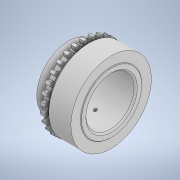
# Autodesk Inventor part: 73. Шестерня третьей передачи
Saved by Autodesk Inventor 2021 (Build 250183000, 183)
## iProperties
Created: 2021-03-26
Part Number: 73. Шестерня третьей передачи
Material: Типовые
Document SubType Name: Modeling
Designer: Данил
Density: 1 g/cm^3
Appearance: По умолчанию
Author: Данил
Autodesk Inventor part; units mm, degrees
ref_plane "YZ Plane" through (0, 0, 0) normal (1, 0, 0) x (0, 1, 0)
sketch "Эскиз1" plane through (0, 0, 0) normal (0, 0, 1) x (1, 0, 0)
  line L0 (-21.5, 0) -> (21.5, 0)
  line L1 (-21.5, -31.5) -> (-10.9, -32)
  line L2 (-21.5, -31.5) -> (-21.5, -25.6)
  line L3 (-19.9, -24) -> (19.9, -24)
  line L4 (-19.9, -24) -> (-21.5, -25.6)
  line L5 (-10.9, -32) -> (-10.9, -32)
  line L6 (-10.4, -31.5) -> (-10.4, -31.5)
  line L7 (-9.9, -32) -> (-9.9, -40.5)
  arc A0 (-10.4, -31.5) -> (-10.9, -32) centre (-10.4, -32) ccw
  arc A1 (-9.9, -32) -> (-10.4, -31.5) centre (-10.4, -32) ccw
  line L8 (-9.9, -40.5) -> (-4.4, -40.5)
  line L9 (-4.4, -40.5) -> (-4.4, -36.5)
  line L10 (-4.4, -36.5) -> (-1, -36.5)
  line L11 (-1, -36.5) -> (-1, -49.276)
  line L12 (-1, -49.276) -> (21, -49.276)
  line L13 (21, -49.276) -> (21, -30.5)
  line L14 (21.5, -30) -> (21.5, -30)
  line L15 (21.5, -30) -> (21.5, -25.6)
  arc A2 (21.5, -30) -> (21, -30.5) centre (21.5, -30.5) ccw
  line L16 (19.9, -24) -> (21.5, -25.6)
  point P0 (0, 0)
  point P1 (0, 0)
  point P2 (-21.5, -24)
  point P3 (21.5, -24)
  dimension "d0" = 43
  dimension "d1" = 1.6
  dimension "d2" = 45
  dimension "d3" = 48
  dimension "d6" = 63
  dimension "d7" = 64
  dimension "d8" = 1
  dimension "d9" = 0.5
  dimension "d10" = 63
  dimension "d11" = 32.4
  dimension "d12" = 5.5
  dimension "d13" = 3.4
  dimension "d14" = 22
  dimension "d17" = 81
  dimension "d18" = 73
  dimension "d19" = 98.552
  dimension "d20" = 0.5
  dimension "d21" = 60
  dimension "d22" = 1.6
  dimension "d23" = 45
  constraints: 34 end point, 7 perpendicular, 6 point on circle, 6 tangent, 4 horizontal, 4 point on line, 3 centre point, 3 vertical, 2 vertical alignment, 1 coincident, 1 concentric, 1 midpoint
  measures "d0" distance of L0.start L0.end
  measures "d1" distance of L3.start point (-21.5, -24)
  measures "d2" angle of L3 L4
  measures "d3" diameter of L3 L0
  measures "d6" diameter of L1.start L0
  measures "d7" diameter of L1.end L0
  measures "d8" distance between parallel lines of L5 L7
  measures "d9" radius of A0
  measures "d10" diameter of L6 L0
  measures "d11" horizontal distance of L0.end L1.end
  measures "d12" distance between parallel lines of L7 L9
  measures "d13" distance of L9.end L10.end
  measures "d14" distance of L11.end L12.end
  measures "d17" diameter of L8 L0
  measures "d18" diameter of L10 L0
  measures "d19" diameter of L12 L0
  measures "d20" radius of A2
  measures "d21" diameter of L14.end L0
  measures "d22" distance of L3.end point (21.5, -24)
  measures "d23" angle of L3 L16
revolve "Вращение1" add sketch "Эскиз1" angle 360 about axis through (-21.5, 0, 0) along (1, 0, 0)
sketch "Эскиз2" plane through (-9.9, 0, 0) normal (-1, 0, 0) x (0, 0, 1)
  circle A0 centre (0, 0) radius 40.5 projected
  circle A1 centre (0, 0) radius 39 construction
  circle A2 centre (0, 0) radius 37
  arc A3 (-1.515, 40.4717) -> (-2.077, 36.9417) centre (3.6162, 37.8449) ccw
  arc A4 (2.077, 36.9417) -> (1.515, 40.4717) centre (-3.6162, 37.8449) ccw
  line L0 (-2.042, 38.9465) -> (2.042, 38.9465) construction
  line L1 (-1.515, 40.4717) -> (1.515, 40.4717) construction
  arc A5 (-9.8964, 39.2723) -> (-9.7123, 35.7026) centre (-4.3312, 37.7697) ccw
  arc A6 (-5.6489, 36.5662) -> (-6.9327, 39.9022) centre (-11.4056, 36.266) ccw
  arc A7 (-17.8453, 36.3565) -> (-16.923, 32.9031) centre (-12.0893, 36.0439) ccw
  arc A8 (-13.1281, 34.5927) -> (-15.0773, 37.5889) centre (-18.6965, 33.1022) ccw
  arc A9 (-25.0143, 31.8518) -> (-23.3941, 28.6656) centre (-19.3191, 32.7427) ccw
  arc A10 (-20.0334, 31.1073) -> (-22.563, 33.6327) centre (-25.1702, 28.4916) ccw
  arc A11 (-31.09, 25.955) -> (-28.8428, 23.1752) centre (-25.7045, 28.0105) ccw
  arc A12 (-26.0632, 26.2623) -> (-29.0626, 28.2067) centre (-30.5439, 22.6358) ccw
  arc A13 (-35.807, 18.9238) -> (-33.0309, 16.6721) centre (-30.9665, 22.0542) ccw
  arc A14 (-30.9539, 20.2696) -> (-34.292, 21.5478) centre (-34.5827, 15.7907) ccw
  arc A15 (-38.959, 11.0656) -> (-35.7754, 9.4402) centre (-34.8751, 15.1339) ccw
  arc A16 (-34.4918, 13.391) -> (-38.0227, 13.9472) centre (-37.1101, 8.2555) ccw
  arc A17 (-40.4083, 2.7238) -> (-36.9564, 1.7958) centre (-37.2596, 7.5523) ccw
  arc A18 (-36.5222, 5.9271) -> (-40.0916, 5.7371) centre (-38.0156, 0.3595) ccw
  arc A19 (-40.0916, -5.7371) -> (-36.5222, -5.9271) centre (-38.0156, -0.3595) ccw
  arc A20 (-36.9564, -1.7958) -> (-40.4083, -2.7238) centre (-37.2596, -7.5523) ccw
  arc A21 (-38.0227, -13.9472) -> (-34.4918, -13.391) centre (-37.1101, -8.2555) ccw
  arc A22 (-35.7754, -9.4402) -> (-38.959, -11.0656) centre (-34.8751, -15.1339) ccw
  arc A23 (-34.292, -21.5478) -> (-30.9539, -20.2696) centre (-34.5827, -15.7907) ccw
  arc A24 (-33.0309, -16.6721) -> (-35.807, -18.9238) centre (-30.9665, -22.0542) ccw
  arc A25 (-29.0626, -28.2067) -> (-26.0632, -26.2623) centre (-30.5439, -22.6358) ccw
  arc A26 (-28.8428, -23.1752) -> (-31.09, -25.955) centre (-25.7045, -28.0105) ccw
  arc A27 (-22.563, -33.6327) -> (-20.0334, -31.1073) centre (-25.1702, -28.4916) ccw
  arc A28 (-23.3941, -28.6656) -> (-25.0143, -31.8518) centre (-19.3191, -32.7427) ccw
  arc A29 (-15.0773, -37.5889) -> (-13.1281, -34.5927) centre (-18.6965, -33.1022) ccw
  arc A30 (-16.923, -32.9031) -> (-17.8453, -36.3565) centre (-12.0893, -36.0439) ccw
  arc A31 (-6.9327, -39.9022) -> (-5.6489, -36.5662) centre (-11.4056, -36.266) ccw
  arc A32 (-9.7123, -35.7026) -> (-9.8964, -39.2723) centre (-4.3312, -37.7697) ccw
  arc A33 (1.515, -40.4717) -> (2.077, -36.9417) centre (-3.6162, -37.8449) ccw
  arc A34 (-2.077, -36.9417) -> (-1.515, -40.4717) centre (3.6162, -37.8449) ccw
  arc A35 (9.8964, -39.2723) -> (9.7123, -35.7026) centre (4.3312, -37.7697) ccw
  arc A36 (5.6489, -36.5662) -> (6.9327, -39.9022) centre (11.4056, -36.266) ccw
  arc A37 (17.8453, -36.3565) -> (16.923, -32.9031) centre (12.0893, -36.0439) ccw
  arc A38 (13.1281, -34.5927) -> (15.0773, -37.5889) centre (18.6965, -33.1022) ccw
  arc A39 (25.0143, -31.8518) -> (23.3941, -28.6656) centre (19.3191, -32.7427) ccw
  arc A40 (20.0334, -31.1073) -> (22.563, -33.6327) centre (25.1702, -28.4916) ccw
  arc A41 (31.09, -25.955) -> (28.8428, -23.1752) centre (25.7045, -28.0105) ccw
  arc A42 (26.0632, -26.2623) -> (29.0626, -28.2067) centre (30.5439, -22.6358) ccw
  arc A43 (35.807, -18.9238) -> (33.0309, -16.6721) centre (30.9665, -22.0542) ccw
  arc A44 (30.9539, -20.2696) -> (34.292, -21.5478) centre (34.5827, -15.7907) ccw
  arc A45 (38.959, -11.0656) -> (35.7754, -9.4402) centre (34.8751, -15.1339) ccw
  arc A46 (34.4918, -13.391) -> (38.0227, -13.9472) centre (37.1101, -8.2555) ccw
  arc A47 (40.4083, -2.7238) -> (36.9564, -1.7958) centre (37.2596, -7.5523) ccw
  arc A48 (36.5222, -5.9271) -> (40.0916, -5.7371) centre (38.0156, -0.3595) ccw
  arc A49 (40.0916, 5.7371) -> (36.5222, 5.9271) centre (38.0156, 0.3595) ccw
  arc A50 (36.9564, 1.7958) -> (40.4083, 2.7238) centre (37.2596, 7.5523) ccw
  arc A51 (38.0227, 13.9472) -> (34.4918, 13.391) centre (37.1101, 8.2555) ccw
  arc A52 (35.7754, 9.4402) -> (38.959, 11.0656) centre (34.8751, 15.1339) ccw
  arc A53 (34.292, 21.5478) -> (30.9539, 20.2696) centre (34.5827, 15.7907) ccw
  arc A54 (33.0309, 16.6721) -> (35.807, 18.9238) centre (30.9665, 22.0542) ccw
  arc A55 (29.0626, 28.2067) -> (26.0632, 26.2623) centre (30.5439, 22.6358) ccw
  arc A56 (28.8428, 23.1752) -> (31.09, 25.955) centre (25.7045, 28.0105) ccw
  arc A57 (22.563, 33.6327) -> (20.0334, 31.1073) centre (25.1702, 28.4916) ccw
  arc A58 (23.3941, 28.6656) -> (25.0143, 31.8518) centre (19.3191, 32.7427) ccw
  arc A59 (15.0773, 37.5889) -> (13.1281, 34.5927) centre (18.6965, 33.1022) ccw
  arc A60 (16.923, 32.9031) -> (17.8453, 36.3565) centre (12.0893, 36.0439) ccw
  arc A61 (6.9327, 39.9022) -> (5.6489, 36.5662) centre (11.4056, 36.266) ccw
  arc A62 (9.7123, 35.7026) -> (9.8964, 39.2723) centre (4.3312, 37.7697) ccw
  point P0 (0, 0)
  point P1 (0, 38.9465)
  point P2 (0, 40.4717)
  point P3 (-10.0948, 37.6709)
  point P4 (-6.1001, 38.52)
  point P5 (-17.7064, 34.7488)
  point P6 (-13.9755, 36.41)
  point P7 (-24.5442, 30.3081)
  point P8 (-21.2402, 32.7086)
  point P9 (-30.3093, 24.5428)
  point P10 (-27.5765, 27.5778)
  point P11 (-34.7497, 17.7048)
  point P12 (-32.7077, 21.2417)
  point P13 (-37.6713, 10.0931)
  point P14 (-36.4093, 13.9772)
  point P15 (-38.9466, 2.0402)
  point P16 (-38.5197, 6.1018)
  point P17 (-38.5197, -6.1018)
  point P18 (-38.9466, -2.0402)
  point P19 (-36.4093, -13.9772)
  point P20 (-37.6713, -10.0931)
  point P21 (-32.7077, -21.2417)
  point P22 (-34.7497, -17.7048)
  point P23 (-27.5765, -27.5778)
  point P24 (-30.3093, -24.5428)
  point P25 (-21.2402, -32.7086)
  point P26 (-24.5442, -30.3081)
  point P27 (-13.9755, -36.41)
  point P28 (-17.7064, -34.7488)
  point P29 (-6.1001, -38.52)
  point P30 (-10.0948, -37.6709)
  point P31 (2.042, -38.9465)
  point P32 (-2.042, -38.9465)
  point P33 (10.0948, -37.6709)
  point P34 (6.1001, -38.52)
  point P35 (17.7064, -34.7488)
  point P36 (13.9755, -36.41)
  point P37 (24.5442, -30.3081)
  point P38 (21.2402, -32.7086)
  point P39 (30.3093, -24.5428)
  point P40 (27.5765, -27.5778)
  point P41 (34.7497, -17.7048)
  point P42 (32.7077, -21.2417)
  point P43 (37.6713, -10.0931)
  point P44 (36.4093, -13.9772)
  point P45 (38.9466, -2.0402)
  point P46 (38.5197, -6.1018)
  point P47 (38.5197, 6.1018)
  point P48 (38.9466, 2.0402)
  point P49 (36.4093, 13.9772)
  point P50 (37.6713, 10.0931)
  point P51 (32.7077, 21.2417)
  point P52 (34.7497, 17.7048)
  point P53 (27.5765, 27.5778)
  point P54 (30.3093, 24.5428)
  point P55 (21.2402, 32.7086)
  point P56 (24.5442, 30.3081)
  point P57 (13.9755, 36.41)
  point P58 (17.7064, 34.7488)
  point P59 (6.1001, 38.52)
  point P60 (10.0948, 37.6709)
  point P61 (5.6489, 36.5662)
  point P62 (6.9327, 39.9022)
  dimension "d25" = 78
  dimension "d26" = 3.5
  dimension "d27" = 4.084
  dimension "d28" = 5.7645
  dimension "d29" = 3.53
  dimension "d32" = 360
  constraints: 186 point on circle, 62 centre point, 4 end point, 2 coincident, 2 midpoint, 2 vertical alignment, 1 horizontal alignment, 301 other
  measures "d25" diameter of A1
  measures "d26" radial gap between concentric circles of A2 A0
  measures "d27" distance of L0.start L0.end
  measures "d28" radius of A4
  measures "d29" vertical distance of A2.end L1.end
extrude "Выдавливание1" cut sketch "Эскиз2" against normal up to surface (8.9 mm away) contours A61 A2 A4 A0
pattern_circular "Круговой массив1" count 30 over 360 about axis through (10, 0, 0) along (-1, 0, 0) of "Выдавливание1"
ref_plane "РабПлоскость1" through (0, 40.5, 0) normal (0, 1, 0) x (-1, 0, 0)
sketch "Эскиз3" plane through (0, 40.5, 0) normal (0, 1, 0) x (-1, 0, 0)
  line L0 (4.4, -2.1482) -> (9.9, -2.1482) projected
  line L1 (4.4, 2.1482) -> (9.9, 2.1482) projected
  line L2 (9.9, -2.1482) -> (9.9, -1.515) projected
  line L3 (9.9, -1.515) -> (9.9, 1.515) projected
  line L4 (9.9, 1.515) -> (9.9, 2.1482) projected
  line L5 (9.9, -32) -> (9.9, 32) projected
  line L6 (9.9, 0) -> (8.2516, -2.1482)
  line L7 (4.4, -2.1482) -> (9.9, -2.1482) projected
  line L8 (9.9, 0) -> (8.2516, 2.1482)
  line L9 (4.4, 2.1482) -> (9.9, 2.1482) projected
  point P0 (0, 0)
  point P1 (9.9, -2.077)
  point P2 (9.9, 2.077)
  dimension "d40" = 105
  constraints: 4 end point, 2 point on line, 1 vertical alignment, 2 other
  measures "d40" angle of L6 L8
extrude "Выдавливание2" cut sketch "Эскиз3" against normal up to surface round surface about axis through (-9.9, 0, 0) along (1, 0, 0) radius 37 far side no
pattern_circular "Круговой массив2" count 30 over 360 about axis through (10, 0, 0) along (-1, 0, 0) of "Выдавливание2"
sketch "Эскиз4" plane through (-9.9, 0, 0) normal (-1, 0, 0) x (0, 0, 1)
  arc A0 (0, 37) -> (-7.6927, 36.1915) centre (0, 0) ccw projected
  line L0 (-4.0978, 37.0742) -> (-3.7, 37.116)
  line L1 (-3.7, 37.116) -> (-3.6686, 36.8177)
  line L2 (-4.0978, 37.0742) -> (-4.0664, 36.7759)
  line L3 (0, 0) -> (-3.8989, 37.0951) construction
  point P0 (0, 0)
  point P1 (-3.8676, 36.7973)
  point P2 (-3.8676, 36.7973)
  dimension "d48" = 0.3
  dimension "d49" = 0.4
  constraints: 8 end point, 4 point on circle, 3 perpendicular, 1 midpoint, 1 point on line
  measures "d48" distance of L0.end L1.end
  measures "d49" distance of L0.start L0.end
extrude "Выдавливание3" add sketch "Эскиз4" against normal up to surface (5.5 mm away)
pattern_circular "Круговой массив3" count 3 over 24 about axis through (-9.9, 0, 0) along (1, 0, 0) of "Выдавливание3"
pattern_circular "Круговой массив4" count 2 over 12 about axis through (-9.9, 0, 0) along (-1, 0, 0) of "Выдавливание3"
mirror "Зеркальное отражение1" about plane through (0, 0, 0) normal (0, 1, 0) of "Круговой массив3", "Круговой массив4", "Выдавливание3"
sketch "Эскиз5" plane through (0, 0, 0) normal (0, 0, 1) x (1, 0, 0)
  line L0 (-4.4, 40.5) -> (-9.9, 40.5) projected
  line L1 (-9.4081, 40.5) -> (-9.9, 37)
  line L2 (-9.9, 36.1915) -> (-9.9, 39.615) projected
  line L3 (-9.9, 0) -> (0, 0)
  line L4 (-9.9, 37) -> (-9.9, 40.5) projected
  dimension "d58" = 8
  constraints: 4 end point, 1 horizontal, 1 point on line, 1 vertical alignment
  measures "d58" angle of L2 L1
revolve "Вращение2" cut sketch "Эскиз5" angle 360 about axis through (-9.9, 0, 0) along (1, 0, 0)
ref_plane "РабПлоскость2" through (0, 0, 8) normal (0, 0, 1) x (1, 0, 0)
sketch "Эскиз6" plane through (0, 0, 8) normal (0, 0, 1) x (1, 0, 0)
  line L0 (-1, 36.5) -> (-4.4, 36.5) projected
  line L1 (-10.9, 32) -> (-21.5, 31.5) projected
  line L2 (-2.7, 36.5) -> (-2.7, 11.5)
  line L3 (-2.7, 11.5) -> (-1.2, 11.5)
  line L4 (-1.2, 11.5) -> (-1.2, 31.5)
  line L5 (-1, 36.5) -> (-1, -36.5) projected
  line L6 (-1.2, 31.5) -> (-1.1, 31.5)
  line L7 (-1.1, 31.5) -> (-1.1, 36.5)
  point P0 (0, 0)
  dimension "d61" = 25
  dimension "d62" = 3.2
  dimension "d63" = 3
  constraints: 10 end point, 2 perpendicular, 1 horizontal, 1 horizontal alignment, 1 midpoint, 1 parallel, 1 point on line, 1 vertical
  measures "d61" distance of L2.start L2.end
  measures "d62" diameter of L7 L2
  measures "d63" diameter of L4 L2
revolve "Вращение3" cut sketch "Эскиз6" angle 360 about axis through (-2.7, 36.5, 8) along (0, -1, 0)
pattern_circular "Круговой массив5" count 2 over 360 about axis through (0, 0, 0) along (-1, 0, 0) of "Вращение3"
sketch "Эскиз9" plane through (-21.5, 0, 0) normal (-1, 0, 0) x (0, 0, 1)
  circle A0 centre (0, 0) radius 23 construction
  circle A1 centre (0, 23) radius 16.5
  dimension "d76" = 46
  dimension "d77" = 33
  constraints: 2 vertical alignment, 1 centre point, 1 coincident, 2 other
  measures "d77" diameter of A1
sketch "Эскиз10" plane through (0, 0, 0) normal (0, 0, 1) x (1, 0, 0)
  line L0 (-21.5, 39.5) -> (-21.5, 6.5) projected
  line L1 (-21.5, 2.5) -> (-21.5, 4.5) construction
  line L2 (-21.5, 4.5) -> (-21.0681, 6.1118)
  arc A0 (-21.0681, 6.1118) -> (-21.0681, 6.8882) centre (-22.517, 6.5) ccw
  line L3 (-21.0681, 6.8882) -> (-21.5, 8.5)
  line L4 (-21.5, 8.5) -> (-21.5, 10.5) construction
  line L5 (-21.5, 4.5) -> (-21.5, 8.5)
  line L6 (-21.5, 31.5) -> (-21.5, -31.5) projected
  point P0 (0, 0)
  dimension "d78" = 15
  dimension "d79" = 15
  dimension "d80" = 1.5
  dimension "d81" = 4
  dimension "d82" = 2
  dimension "d83" = 2
  constraints: 10 end point, 2 point on circle, 2 tangent, 2 vertical, 1 centre point, 1 collinear, 1 horizontal alignment, 1 point on line, 1 vertical alignment
  measures "d78" angle of L4 L3
  measures "d79" angle of L1 L2
  measures "d80" radius of A0
  measures "d81" distance of L1.end L3.end
  measures "d82" distance of L3.end L4.end
  measures "d83" distance of L1.start L1.end
sweep "Сдвиг2" cut profiles "Эскиз10" path "Эскиз9"
pattern_circular "Круговой массив6" count 2 over 360 about axis through (0, 0, 0) along (-1, 0, 0) of "Сдвиг2"
sketch "Эскиз11" plane through (0, 0, 0) normal (0, 0, 1) x (1, 0, 0)
  line L0 (-1, 49.276) -> (-1, -49.276) projected
  line L1 (21, 49.276) -> (21, -49.276) projected
  line L2 (-1, 49.276) -> (21, 49.276)
  line L3 (21, 49.276) -> (21, 40)
  line L4 (21, 40) -> (-1, 40)
  line L5 (-1, 40) -> (-1, 49.276)
  line L6 (-1, 0) -> (21, 0)
  point P0 (0, 0)
  point P1 (-1, 40)
  dimension "d89" = 80
  constraints: 10 end point, 2 midpoint, 2 parallel, 1 horizontal, 1 perpendicular, 1 point on line
  measures "d89" diameter of L4 L6
revolve "Вращение4" cut sketch "Эскиз11" angle 360 about axis through (-1, 0, 0) along (1, 0, 0) contours L2 L1 L4 L0
